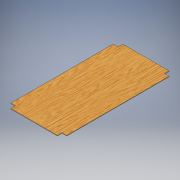
# Autodesk Inventor part: Wooden Rack Plate
Saved by Autodesk Inventor 2019.4 (Build 234330000, 330)
## iProperties
Created: 2020-02-27
Part Number: Wooden Rack Plate
Material: Plywood, Finish
Document SubType Name: Modeling
Designer: admin
Density: 0.552 g/cm^3
Appearance: Plywood - New
Author: admin
Autodesk Inventor part; units mm, degrees
ref_plane "YZ Plane" through (0, 0, 0) normal (1, 0, 0) x (0, 1, 0)
ref_plane "XZ Plane" through (0, 0, 0) normal (0, 1, 0) x (-1, 0, 0)
ref_plane "XY Plane" through (0, 0, 0) normal (0, 0, 1) x (1, 0, 0)
sketch "Sketch1" plane through (0, 0, 0) normal (0, 1, 0) x (-1, 0, 0)
  line L0 (-250, 500) -> (-208, 500) construction
  line L1 (250, 500) -> (250, 458) construction
  line L2 (250, -500) -> (208, -500) construction
  line L3 (-250, -500) -> (-250, -458) construction
  line L4 (-250, 500) -> (250, -500) construction
  line L5 (250, 500) -> (-250, -500) construction
  line L6 (250, 500) -> (208, 500) construction
  line L7 (208, 500) -> (208, 458)
  line L8 (208, 458) -> (250, 458)
  line L9 (250, 458) -> (250, 500) construction
  line L10 (-250, 500) -> (-208, 500) construction
  line L11 (-208, 500) -> (-208, 458)
  line L12 (-208, 458) -> (-250, 458)
  line L13 (-250, 458) -> (-250, 500) construction
  line L14 (-250, -500) -> (-208, -500) construction
  line L15 (-208, -500) -> (-208, -458)
  line L16 (-208, -458) -> (-250, -458)
  line L17 (-250, -458) -> (-250, -500) construction
  line L18 (250, -500) -> (208, -500) construction
  line L19 (208, -500) -> (208, -458)
  line L20 (208, -458) -> (250, -458)
  line L21 (250, -458) -> (250, -500) construction
  line L22 (208, 500) -> (250, 500) construction
  line L23 (250, 458) -> (250, -458)
  line L24 (-208, 500) -> (208, 500)
  line L25 (-250, 458) -> (-250, 500) construction
  line L26 (-250, -458) -> (-250, 458)
  line L27 (-208, -500) -> (-250, -500) construction
  line L28 (208, -500) -> (-208, -500)
  line L29 (250, -458) -> (250, -500) construction
  point P0 (0, 0)
  dimension "d0" = 500
  dimension "d1" = 1000
  dimension "d2" = 42
  dimension "d3" = 42
  dimension "d4" = 42
  dimension "d5" = 42
  dimension "d6" = 42
  dimension "d7" = 42
  dimension "d8" = 42
  dimension "d9" = 42
  constraints: 60 end point, 26 parallel, 13 perpendicular, 7 horizontal, 2 midpoint
  measures "d0" distance of L2.start L3.start
  measures "d1" distance of L1.start L2.start
  measures "d2" distance of L1.end L7.end
  measures "d3" distance of L7.end L6.end
  measures "d4" distance of L11.end L12.end
  measures "d5" distance of L0.end L11.end
  measures "d6" distance of L3.end L15.end
  measures "d7" distance of L15.end L14.end
  measures "d8" distance of L19.end L20.end
  measures "d9" distance of L2.end L19.end
extrude "Extrusion1" add sketch "Sketch1" along normal blind 5
body "Solid1"
